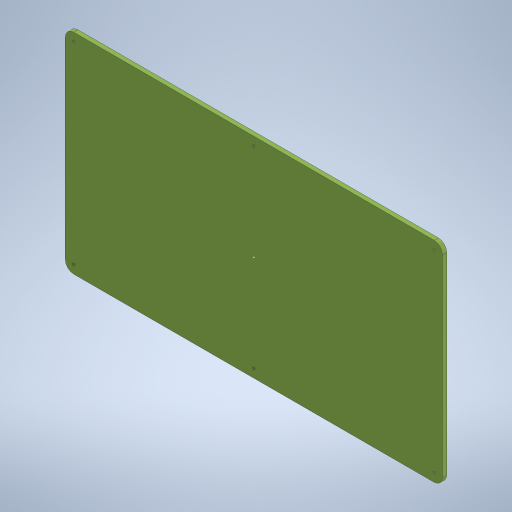
# Autodesk Inventor part: base
Saved by Autodesk Inventor 2024 (Build 280153000, 153)
## iProperties
Created: 2023-12-01
Part Number: base
Material: Generic
Document SubType Name: Modeling
Designer: cnola
Density: 1 g/cm^3
Appearance: Default
Author: cnola
Autodesk Inventor part; units mm, degrees
ref_plane "YZ Plane" through (0, 0, 0) normal (1, 0, 0) x (0, 1, 0)
ref_plane "XZ Plane" through (0, 0, 0) normal (0, 1, 0) x (-1, 0, 0)
ref_plane "XY Plane" through (0, 0, 0) normal (0, 0, 1) x (1, 0, 0)
sketch "Sketch1" plane through (0, 0, 0) normal (0, 0, 1) x (1, 0, 0)
  point P0 (0, 0)
sketch "Sketch2" plane through (0, 0, 0) normal (0, 0, 1) x (1, 0, 0)
  line L0 (215, -125) -> (-215, -125)
  line L1 (-225, -115) -> (-225, 115)
  line L2 (-215, 125) -> (215, 125)
  line L3 (225, 115) -> (225, -115)
  line L4 (225, 0) -> (225, 25)
  line L5 (225, 25) -> (225, 0)
  arc A0 (225, 115) -> (215, 125) centre (215, 115) ccw
  arc A1 (-215, 125) -> (-225, 115) centre (-215, 115) ccw
  arc A2 (-225, -115) -> (-215, -125) centre (-215, -115) ccw
  arc A3 (215, -125) -> (225, -115) centre (215, -115) ccw
  line L6 (-232.4948, 131.6024) -> (-218.9232, 118.3976) construction
  line L7 (-182.3, 125) -> (-145.3, 125)
  line L8 (-145.3, -125) -> (-182.3, -125)
  line L9 (145.3, -125) -> (182.3, -125)
  line L10 (145.3, 125) -> (182.3, 125)
  line L11 (-225, 125) -> (-182.3, 125)
  point P0 (0, 0)
  point P1 (0, 0)
  point P2 (-225.709, 125)
  dimension "d13" = 10
  dimension "d14" = 10
  dimension "d15" = 10
  dimension "d16" = 10
  dimension "d67" = 450
  constraints: 24 end point, 8 point on circle, 8 tangent, 4 centre point, 3 horizontal, 3 point on line, 2 midpoint, 2 parallel, 2 perpendicular, 1 coincident, 1 collinear
  measures "d13" radius of A0
  measures "d14" radius of A1
  measures "d15" radius of A2
  measures "d16" radius of A3
  measures "d67" distance between parallel lines of L3 L1
extrude "Extrusion2" add sketch "Sketch2" along normal blind 5
sketch "Sketch10" plane through (0, 0, 5) normal (0, 0, 1) x (1, 0, 0)
  point P0 (0, 0)
sketch "Sketch11" plane through (0, 0, 5) normal (0, 0, 1) x (1, 0, 0)
  line L0 (-225, 115) -> (-225, -115) projected
  line L1 (215, 125) -> (-215, 125) projected
  point P0 (0, 0)
  point P1 (-215, 115)
  point P2 (-215, 0)
  point P3 (-215, -115)
  point P4 (0, 115)
  point P5 (0, 0)
  point P6 (0, -115)
  point P7 (215, 115)
  point P8 (215, 0)
  point P9 (215, -115)
  dimension "d77" = 10
  dimension "d78" = 10
  dimension "d81" = 115
  dimension "d84" = 215
  constraints: 1 horizontal, 1 vertical, 8 other
  measures "d77" distance from line of L0 point (-215, 115)
  measures "d78" distance from line of point (-215, 115) L1
  measures "d81" distance of point (-215, 115) point (-215, 0)
  measures "d84" distance of point (-215, 115) point (0, 115)
hole "Hole2" at (-215, 115, 5) at (0, 115, 5) at (215, 115, 5) at (215, -115, 5) at (-215, -115, 5) at (0, -115, 5) direction (0, 0, -1) diameter 2.459 end through all thread size "M3x0.5" class "6H" standard "ISO Metric profile"
body "Solid2"
